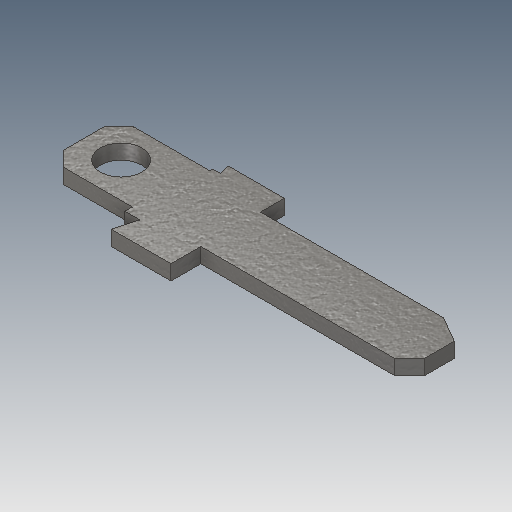
# Autodesk Inventor part: PlacaTerraPlug
Saved by Autodesk Inventor 2020.3 (Build 243373000, 373)
## iProperties
Created: 2015-09-19
Part Number: PlacaTerraPlug
Material: Steel, Galvanized
Document SubType Name: Sheet Metal
Designer: Elvis Mayk
Density: 7.85 g/cm^3
Sheet Metal Rule: Default_mm
Appearance: Galvanized
Author: Elvis Mayk
Autodesk Inventor part; units mm, degrees
ref_plane "YZ Plane" through (0, 0, 0) normal (1, 0, 0) x (0, 1, 0)
ref_plane "XZ Plane" through (0, 0, 0) normal (0, 1, 0) x (-1, 0, 0)
ref_plane "XY Plane" through (0, 0, 0) normal (0, 0, 1) x (1, 0, 0)
sketch "Sketch1" plane through (0, 0, 0) normal (0, 1, 0) x (-1, 0, 0)
  line L0 (-4.1, 2.85) -> (-3.1, 2.85)
  line L1 (-3.1, 2.85) -> (-3.1, 2.35)
  line L2 (-3.1, 2.35) -> (2.5, 2.35)
  line L3 (2.5, 2.35) -> (2.5, -2.35)
  line L4 (-4.1, 2.85) -> (-3.6981, 4.35)
  line L5 (-3.6981, 4.35) -> (-7.6981, 4.35)
  line L6 (-7.6981, 4.35) -> (-7.6981, 2.35)
  line L7 (-7.6981, 2.35) -> (-20.6981, 2.35)
  line L8 (-20.6981, 2.35) -> (-21.6981, 1.35)
  line L9 (-21.6981, 1.35) -> (-21.6981, -0.65)
  line L10 (-21.6981, -0.65) -> (-19.966, -1.65)
  line L11 (-19.966, -1.65) -> (-7.6981, -1.65)
  line L12 (-7.6981, -1.65) -> (-7.6981, -3.25)
  line L13 (-7.6981, -3.25) -> (-3.9124, -3.25)
  line L14 (-3.9124, -3.25) -> (-4.1, -2.55)
  line L15 (-4.1, -2.55) -> (-3.6, -2.55)
  line L16 (-3.6, -2.55) -> (-3.6, -2.35)
  line L17 (-3.6, -2.35) -> (2.5, -2.35)
  circle A0 centre (0, 0) radius 1.4
  dimension "d1" = 4
  dimension "d2" = 2
  dimension "d3" = 75
  dimension "d4" = 4.7
  dimension "d5" = 5.6
  dimension "d6" = 1
  dimension "d7" = 0.5
  dimension "d8" = 75
  dimension "d9" = 7.6
  dimension "d10" = 2
  dimension "d11" = 0.5
  dimension "d12" = 0.2
  dimension "d13" = 2.8
  dimension "d14" = 2.5
  dimension "d15" = 2.35
  dimension "d17" = 0
  dimension "d18" = 0
  dimension "d19" = 4
  dimension "d20" = 0
  dimension "d21" = 0
  dimension "d23" = 2
  dimension "d24" = 60
  dimension "d25" = 45
  dimension "d26" = 14
  dimension "d27" = 1
  measures "d1" distance of L4.end L5.end
  measures "d2" distance of L5.end L6.end
  measures "d3" angle of L0 L4
  measures "d4" distance of L2.end L3.end
  measures "d5" distance from line of L3 L1.end
  measures "d6" distance of L0.start L0.end
  measures "d7" distance of L14.end L15.end
  measures "d8" angle of L15 L14
  measures "d9" distance between parallel lines of L13 L5
  measures "d10" distance between parallel lines of L5 L2
  measures "d11" distance of L0.end L1.end
  measures "d12" distance between parallel lines of L15 L17
  measures "d13" diameter of A0
  measures "d14" distance from line of L3 A0.centre
  measures "d15" distance from line of A0.centre L17
  measures "d17" distance of point (0, 0) A0.centre
  measures "d18" distance of point (0, 0) A0.centre
  measures "d19" distance between parallel lines of L11 L7
  measures "d20" distance between parallel lines of L12 L6
  measures "d21" horizontal distance of L14.end L0.start
  measures "d23" distance of L8.end L9.end
  measures "d24" angle of L9 L10
  measures "d25" angle of L8 L7
  measures "d26" distance between parallel lines of L6 L9
  measures "d27" horizontal distance of L7.end L8.end
extrude "Plate1" add sketch "Sketch1" along normal blind 1
chamfer "Corner Chamfer1" distance 1 angle 45 2 edges at (-2.5, 0.5, 2.35) (-2.5, 0.5, -2.35)
equation "\"d8\" = d3"
equation "\"d15\" = 0.5 * d4"
equation "\"d31\" = Thickness"
equation "\"BendRadius\" = Thickness"
equation "\"BendReliefWidth\" = Thickness"
equation "\"BendReliefDepth\" = 0.5 * Thickness"
equation "\"CornerReliefSize\" = 4 * Thickness"
equation "\"MinimumRemnant\" = 2 * Thickness"
equation "\"TransitionRadius\" = BendRadius"
equation "\"JacobiRadiusSize\" = BendRadius"
equation "\"GapSize\" = Thickness"
equation "\"d16\" = BendRadius"
equation "\"Thickness\" = 1"
body "Solid1"
